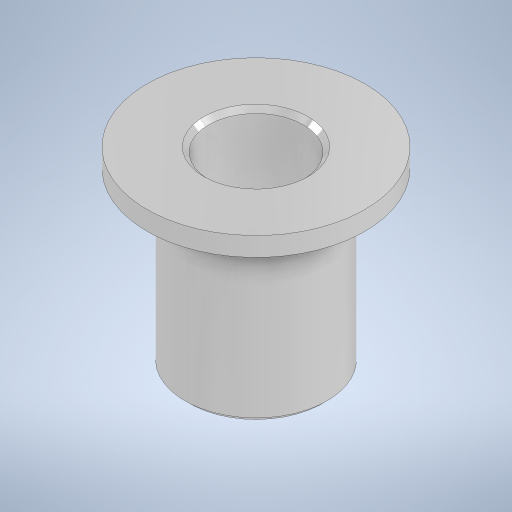
# Autodesk Inventor part: sleeve
Saved by Autodesk Inventor 2023 (Build 270158000, 158)
## iProperties
Created: 2023-06-30
Part Number: sleeve
Material: Алюминий 6061-AHC
Document SubType Name: Modeling
Designer: khrip
Density: 2.7 g/cm^3
Appearance: Алюминий — темный
Author: khrip
Autodesk Inventor part; units mm, degrees
ref_plane "YZ Plane" through (0, 0, 0) normal (1, 0, 0) x (0, 1, 0)
ref_plane "XZ Plane" through (0, 0, 0) normal (0, 1, 0) x (-1, 0, 0)
ref_plane "XY Plane" through (0, 0, 0) normal (0, 0, 1) x (1, 0, 0)
sketch "Эскиз1" plane through (0, 0, 0) normal (1, 0, 0) x (0, 1, 0)
  line L0 (10, -2.5) -> (10, -5.75)
  line L1 (10, -5.75) -> (9, -5.75)
  line L2 (9, -5.75) -> (9, -3.75)
  line L3 (9, -3.75) -> (0, -3.75)
  line L4 (0, -3.75) -> (0, -2.5)
  line L5 (0, -2.5) -> (10, -2.5)
  line L6 (-2, 0) -> (12, 0) projected
  point P0 (0, 0)
  dimension "d0" = 2.5
  dimension "d1" = 3.75
  dimension "d2" = 1
  dimension "d3" = 10
  dimension "d4" = 5.75
  constraints: 12 end point, 5 perpendicular, 1 vertical
  measures "d0" distance from line of L5 point (0, 0)
  measures "d1" distance from line of point (0, 0) L3
  measures "d2" distance between parallel lines of L0 L2
  measures "d3" distance between parallel lines of L4 L0
  measures "d4" distance from line of point (0, 0) L1
revolve "Вращение1" add sketch "Эскиз1" angle 360 about axis through (0, -10, 0) along (0, 1, 0)
chamfer "Фаска1" distance 0.25 angle 45 3 edges at (0, 10, 2.5) (0, 0, 2.5) (0, 0, 3.75)
